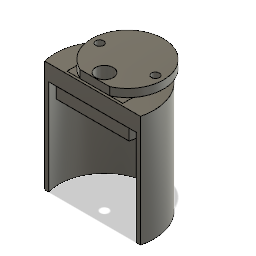
Stepper Motor Holder (Autodesk Fusion 360 design; units mm, degrees)
Autodesk Fusion 360 part; units mm, degrees
sketch "Sketch1" plane through (0, 0, 0) normal (0, 1, 0) x (1, 0, 0)
  circle A0 centre (0, 0) radius 2.5
  line L0 (0, -2.5) -> (0, -7.5) construction
  line L1 (0, -7.5) -> (22.798, -7.5)
  line L2 (0, -7.5) -> (-22.798, -7.5)
  arc A1 (22.798, -7.5) -> (-22.798, -7.5) centre (0, 0) ccw
  dimension "d5" = 5
  dimension "d8" = 5
  dimension "d9" = 24
  constraint coincident A0.centre A1.centre
  constraint coincident A0 L0.start
  constraint vertical L0
  constraint vertical A0.centre L0.end
  constraint perpendicular L0 L1
  constraint perpendicular L0 L2
  measures "d5" diameter of A0
  measures "d8" distance of L0.start L0.end
  measures "d9" radius of A1
extrude "Extrude1" add sketch "Sketch1" along normal blind 7 makes body 1
sketch "Sketch4" plane through (0, 7, 0) normal (0, 1, 0) x (-1, 0, 0)
  circle A0 centre (0, 0) radius 2.5
  line L0 (22.798, 7.5) -> (-22.798, 7.5)
  arc A1 (-22.798, 7.5) -> (22.798, 7.5) centre (0, 0) ccw construction
  circle A2 centre (0, 0) radius 5.5
  line L1 (30.0754, 7.5148) -> (-30.0754, 7.5148)
  arc A3 (-30.0754, 7.5148) -> (30.0754, 7.5148) centre (0, 0) ccw
  dimension "d12" = 62
  dimension "d13" = 11
  constraint coincident A0.centre A1.centre
  constraint parallel L0 L1
  measures "d12" diameter of A3
  measures "d13" diameter of A2
extrude "Extrude2" add sketch "Sketch4" along normal blind 10 contours L1 A3 bodies 1
sketch "Sketch5" plane through (0, 7, 0) normal (0, -1, 0) x (1, 0, 0)
  arc A0 (-30.0754, 7.5148) -> (30.0754, 7.5148) centre (0, 0) ccw
  line L0 (30.0754, 7.5148) -> (-30.0754, 7.5148)
  arc A1 (-22.798, 7.5) -> (22.798, 7.5) centre (0, 0) ccw
  line L1 (-22.798, 7.5) -> (22.798, 7.5)
  line L2 (-30.0754, 7.5148) -> (30.0754, 7.5148)
  arc A2 (-30.0754, 7.5148) -> (30.0754, 7.5148) centre (0, 0) ccw
  arc A3 (-27.4914, 7.5148) -> (27.4914, 7.5148) centre (0, 0) ccw
  dimension "d18" = 28.5
  constraint coincident A0.centre A1.centre
  constraint coincident A0.start L0.end
  constraint coincident A0.end L0.start
  constraint coincident L0 A3.end
  constraint coincident L0 A3.start
  measures "d18" radius of A3
extrude "Extrude3" add sketch "Sketch5" along normal blind 60 contours A0 L0 L2 A2 A3 bodies 1
sketch "Sketch7" plane through (0, 17, 0) normal (0, 1, 0) x (-1, 0, 0)
  circle A0 centre (0, 0) radius 5.5
  arc A1 (-30.0754, 7.5148) -> (30.0754, 7.5148) centre (0, 0) ccw
  line L0 (30.0754, 7.5148) -> (-30.0754, 7.5148)
  circle A2 centre (0, 0) radius 17.5
  dimension "d21" = 35
  constraint coincident A0.centre A1.centre
  measures "d21" diameter of A2
sketch "Sketch11" plane through (0, 17, 0) normal (0, 1, 0) x (-1, 0, 0)
  circle A0 centre (0, 0) radius 5.5
  arc A1 (-30.0754, 7.5148) -> (30.0754, 7.5148) centre (0, 0) ccw
  line L0 (30.0754, 7.5148) -> (-30.0754, 7.5148)
  line L1 (-17.5, -6) -> (-17.5, 6)
  line L2 (-17.5, 6) -> (17.5, 6)
  line L3 (17.5, 6) -> (17.5, -6)
  line L4 (6, 6) -> (-6, 6)
  line L5 (-6, -6) -> (-6, -18)
  line L6 (-6, -18) -> (6, -18)
  line L7 (6, -18) -> (6, -6)
  line L8 (17.5, -6) -> (6, -6)
  line L9 (-6, -6) -> (-17.5, -6)
  line L10 (17.5, 0) -> (0, 0) construction
  line L11 (0, 0) -> (-17.5, 0) construction
  point P0 (17.5, 0)
  point P1 (0, -18)
  dimension "d30" = 12
  dimension "d31" = 35
  dimension "d32" = 12
  dimension "d33" = 24
  constraint horizontal L8
  constraint vertical L1
  constraint horizontal L2
  constraint vertical L3
  constraint midpoint L3 P0
  constraint horizontal A0.centre L10.start
  constraint horizontal L4
  constraint vertical L5
  constraint horizontal L6
  constraint vertical L7
  constraint coincident L2 L4.start
  constraint midpoint L6 P1
  constraint collinear L8 L9
  constraint coincident P0 L10.start
  constraint coincident A0.centre A1.centre
  constraint midpoint L1 L11.end
  constraint equal L10 L11
  constraint vertical A0.centre P1
  measures "d30" distance of L3.end L2.end
  measures "d31" distance of L3.end L1.start
  measures "d32" distance of L5.end L6.end
  measures "d33" distance of L4.end L5.end
extrude "Extrude8" cut sketch "Sketch11" against normal blind 5 contours L1 L2 L3 L4 L5 L6 L7 L8 L9 bodies 1
sketch "Sketch12" plane through (0, 12, 0) normal (0, 1, 0) x (-1, 0, 0)
  circle A0 centre (0, 0) radius 5.5
  line L0 (-6, -18) -> (6, -18)
  line L1 (6, -18) -> (6, -6)
  line L2 (6, -6) -> (17.5, -6)
  line L3 (17.5, -6) -> (17.5, 6)
  line L4 (17.5, 6) -> (-17.5, 6)
  line L5 (-17.5, 6) -> (-17.5, -6)
  line L6 (-17.5, -6) -> (-6, -6)
  line L7 (-6, -6) -> (-6, -18)
  line L8 (6, -6) -> (6, -18)
  line L9 (-6, -18) -> (-6, -6)
  line L10 (-17.5, -6) -> (-17.5, 6)
  line L11 (17.5, 6) -> (17.5, -6)
  circle A1 centre (0, 0) radius 5.5
  constraint coincident L1.end L2.start
  constraint coincident L0.end L1.start
  constraint coincident L0.start L7.end
  constraint coincident L6.end L7.start
  constraint coincident L5.end L6.start
  constraint coincident L4.end L5.start
  constraint coincident L3.end L4.start
  constraint coincident L2.end L3.start
  constraint concentric A0 A1
extrude "Extrude9" add sketch "Sketch12" along normal blind 5 separate body makes body 2
sketch "Sketch13" plane through (0, 17, 0) normal (0, 1, 0) x (-1, 0, 0)
  circle A0 centre (0, 0) radius 5.5
  line L0 (-17.5, -6) -> (-6, -6)
  line L1 (-6, -6) -> (-6, -18)
  line L2 (-6, -18) -> (6, -18)
  line L3 (6, -18) -> (6, -6)
  line L4 (6, -6) -> (17.5, -6)
  line L5 (17.5, -6) -> (17.5, 6)
  line L6 (17.5, 6) -> (-17.5, 6)
  line L7 (-17.5, 6) -> (-17.5, -6)
  circle A1 centre (0.013, -14.5) radius 22.5
  line L8 (0, 0) -> (0, -10) construction
  line L9 (0.013, -14.5) -> (-17.487, -14.5) construction
  line L10 (0.013, -14.5) -> (17.513, -14.5) construction
  circle A2 centre (17.513, -14.5) radius 2.5
  circle A3 centre (-17.487, -14.5) radius 2.5
  point P0 (0, 5.5)
  point P1 (0, 8)
  dimension "d38" = 2.5
  dimension "d40" = 22.5
  dimension "d41" = 17.5
  dimension "d42" = 5
  constraint coincident A0 P0
  constraint coincident A1 P1
  constraint vertical P0 P1
  constraint vertical A0.centre P1
  constraint coincident A0.centre L8.start
  constraint vertical L8
  constraint coincident A1.centre L9.start
  constraint horizontal L9
  constraint parallel L9 L10
  constraint equal L9 L10
  constraint coincident L10.end A2.centre
  constraint coincident L9.end A3.centre
  constraint equal A2 A3
  measures "d38" distance of P0 P1
  measures "d40" radius of A1
  measures "d41" distance of A1.centre L10.end
  measures "d42" diameter of A2
extrude "Extrude10" add sketch "Sketch13" along normal blind 5 separate body contours L0 L1 L2 L3 L4 L5 L6 L7 A1 | L0 L1 L2 L3 L4 L5 L7 A1 makes body 3
sketch "Sketch14" plane through (0, 17, 0) normal (0, 1, 0) x (-1, 0, 0)
  line L0 (6, -6) -> (6, -18)
  line L1 (6, -18) -> (-6, -18)
  line L2 (-6, -18) -> (-6, -6)
  line L3 (-6, -6) -> (-17.5, -6)
  line L4 (-17.5, -6) -> (-17.5, 6)
  line L5 (-17.5, 6) -> (17.5, 6)
  line L6 (17.5, 6) -> (17.5, -6)
  line L7 (17.5, -6) -> (6, -6)
  arc A0 (-30.0754, 7.5148) -> (30.0754, 7.5148) centre (0, 0) ccw
  line L8 (30.0754, 7.5148) -> (-30.0754, 7.5148)
  circle A1 centre (17.5, -14.5) radius 3.3879
  circle A2 centre (-17.5131, -14.5) radius 3.3879
  constraint equal A1 A2
extrude "Extrude11" cut sketch "Sketch14" against normal blind 3 contours A1 | A2 bodies 1
combine "Combine1" operation add target body 2 tool bodies 3
sketch "Sketch16" plane through (0, 17, 0) normal (0, 1, 0) x (-1, 0, 0)
  line L0 (17.5, -0.3418) -> (17.5, 6)
  line L1 (17.5, 6) -> (9.2866, 6)
  circle A0 centre (13, 0) radius 2.5
  circle A1 centre (-13, 0) radius 2.5
  line L2 (0, 0) -> (13, 0) construction
  line L3 (0, 0) -> (-13, 0) construction
  arc A2 (17.5, -0.3418) -> (9.2866, 6) centre (0.013, -14.5) ccw
  dimension "d47" = 5
  constraint coincident L2.start L3.start
  constraint coincident A0.centre L2.end
  constraint horizontal L2
  constraint coincident A1.centre L3.end
  constraint parallel L2 L3
  constraint equal L2 L3
  constraint equal A0 A1
  measures "d47" diameter of A0
extrude "Extrude12" cut sketch "Sketch16" against normal blind 20 contours A0 | A1 bodies 1
sketch "Sketch17" plane through (0, 17, 0) normal (0, 1, 0) x (-1, 0, 0)
  circle A0 centre (-13, 0) radius 2.2361
  circle A1 centre (13, 0) radius 2.5146
extrude "Extrude13" cut sketch "Sketch16" sketch "Sketch17" against normal blind 5 contours A1 of sketch 2 contours A1 bodies 2
